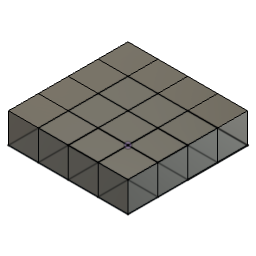
1m cubes v1 (Autodesk Fusion 360 design; units mm, degrees)
Autodesk Fusion 360 part; units mm, degrees
sketch "Sketch1" plane through (0, 0, 0) normal (0, 1, 0) x (1, 0, 0)
  line L0 (0, 0) -> (1000, 0)
  line L1 (1000, 0) -> (1000, 1000)
  line L2 (1000, 1000) -> (0, 1000)
  line L3 (0, 1000) -> (0, 0)
  line L4 (0, 0) -> (-1000, 0)
  line L5 (-1000, 0) -> (-1000, -1000)
  line L6 (-1000, -1000) -> (0, -1000)
  line L7 (0, -1000) -> (0, 0)
  line L8 (1000, 1000) -> (-1000, 1000)
  line L9 (-1000, 1000) -> (-1000, -1000)
  line L10 (-1000, -1000) -> (1000, -1000)
  line L11 (1000, -1000) -> (1000, 1000)
  line L12 (0, 0) -> (2000, 0)
  line L13 (2000, 0) -> (2000, 2000)
  line L14 (2000, 2000) -> (0, 2000)
  line L15 (0, 2000) -> (0, 0)
  line L16 (2000, 2000) -> (-2000, 2000)
  line L17 (-2000, 2000) -> (-2000, -2000)
  line L18 (-2000, -2000) -> (2000, -2000)
  line L19 (2000, -2000) -> (2000, 2000)
  line L20 (0, 0) -> (-2000, 0)
  line L21 (0, 0) -> (0, -2000)
  line L22 (-1000, -1000) -> (-2000, -1000)
  line L23 (-1000, -1000) -> (-1000, -2000)
  line L24 (1000, -1000) -> (1000, -2000)
  line L25 (1000, -1000) -> (2000, -1000)
  line L26 (1000, 1000) -> (2000, 1000)
  line L27 (1000, 1000) -> (1000, 2000)
  line L28 (-1000, 1000) -> (-1000, 2000)
  line L29 (-1000, 1000) -> (-2000, 1000)
  dimension "d1" = 1000
  dimension "d2" = 1000
  dimension "d3" = 1000
  dimension "d4" = 1000
  dimension "d5" = 2000
  dimension "d6" = 2000
  dimension "d7" = 4000
  dimension "d8" = 4000
  constraint horizontal L0
  constraint vertical L1
  constraint horizontal L2
  constraint vertical L3
  constraint coincident L0.start L3.end
  constraint horizontal L4
  constraint vertical L5
  constraint horizontal L6
  constraint vertical L7
  constraint horizontal L8
  constraint vertical L9
  constraint horizontal L10
  constraint vertical L11
  constraint horizontal L12
  constraint vertical L13
  constraint horizontal L14
  constraint vertical L15
  constraint horizontal L16
  constraint vertical L17
  constraint horizontal L18
  constraint vertical L19
  constraint midpoint L17 L20.end
  constraint midpoint L18 L21.end
  constraint coincident L17 L22.end
  constraint perpendicular L17 L22
  constraint coincident L18 L23.end
  constraint perpendicular L18 L23
  constraint coincident L18 L24.end
  constraint perpendicular L18 L24
  constraint coincident L19 L25.end
  constraint perpendicular L19 L25
  constraint midpoint L13 L26.end
  constraint midpoint L14 L27.end
  constraint coincident L16 L28.end
  constraint perpendicular L16 L28
  constraint coincident L17 L29.end
  constraint perpendicular L17 L29
  measures "d1" distance of L0.start L0.end
  measures "d2" distance of L0.start L2.end
  measures "d3" distance of L0.start L4.end
  measures "d4" distance of L0.start L6.end
  measures "d5" distance of L0.start L12.end
  measures "d6" distance of L0.start L14.end
  measures "d7" distance of L13.end L16.end
  measures "d8" distance of L13.end L18.end
extrude "Extrude1" add sketch "Sketch1" along normal blind 1000 contours L16 L17 L28 L29 makes body 1
extrude "Extrude2" add sketch "Sketch1" along normal blind 1000 separate body contours L8 L15 L16 L28 makes body 2
copy_body "CopyPasteBodies1" bodies 2 1 makes body 3 makes body 4
move_body "Move1" bodies 3 4 to x (1, 0, 0) y (0, 1, 0) z (0, 0, 1) at (2000, 0, 0)
copy_body "CopyPasteBodies2" bodies 4 1 2 3 makes body 5 makes body 6 makes body 7 makes body 8
move_body "Move2" bodies 5 6 7 8 to x (1, 0, 0) y (0, 1, 0) z (0, 0, 1) at (0, 0, 1000)
copy_body "CopyPasteBodies3" bodies 1 2 3 4 6 5 7 8 makes body 9 makes body 10 makes body 11 makes body 12 makes body 13 makes body 14 makes body 15 makes body 16
move_body "Move3" bodies 9 10 11 12 13 14 15 16 to x (1, 0, 0) y (0, 1, 0) z (0, 0, 1) at (0, 0, 2000)
